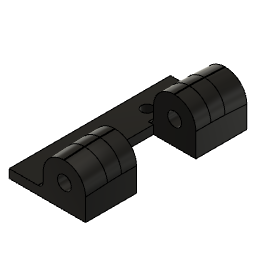
Front mount attachment (Autodesk Fusion 360 design; units mm, degrees)
Autodesk Fusion 360 part; units mm, degrees
box "BoitePrimitive1" add length 25 width 25 height -95 placed x (0, 1, 0) y (-1, 0, 0) z (0, 0, 1) at (25, 0, 0) makes body 1
move_face "DécalerLesFaces3" offset 1.5 1 faces at (16.6667, 25, -63.3333) on bodies 1
sketch "Esquisse8" plane through (0, 0, 0) normal (0, 0, 1) x (1, 0, 0)
  line L0 (0, 0) -> (25, 0)
  line L1 (25, 0) -> (25, 26.5)
  line L2 (25, 26.5) -> (0, 26.5)
  line L3 (0, 26.5) -> (0, 0)
  circle A0 centre (25, 26.5) radius 25 construction
  line L4 (0, 26.5) -> (25, 1.5) construction
  line L5 (25, 26.5) -> (0, 1.5) construction
  point P0 (12.5, 14)
  constraint coincident L1.end L2.start
  constraint coincident L2.end A0
  constraint coincident L2.end L3.start
  constraint coincident A0 L4.end
  constraint coincident L1 L4.end
  constraint coincident L3 L5.end
  constraint perpendicular L4 L5
  constraint midpoint L4 P0
hole "Perçage2" at (12.5, 14, 0) direction (0, 0, -1) diameter 8.2 end through all bodies 1
box "BoitePrimitive2" add length 95 width 20 height 5 placed x (0, 0, -1) y (-1, 0, 0) z (0, 1, 0) at (0, 0, 0) separate body makes body 2
sketch "Esquisse7" plane through (0, 5, 0) normal (0, 1, 0) x (-1, 0, 0)
  line L0 (0, -95) -> (20, -95)
  line L1 (20, -95) -> (20, 0)
  line L2 (20, 0) -> (0, 0)
  line L3 (0, 0) -> (0, -95)
  line L4 (20, -47.5) -> (0, -47.5) construction
  line L5 (20, -95) -> (0, -47.5) construction
  line L6 (0, -47.5) -> (20, 0) construction
  line L7 (0, 0) -> (20, -47.5) construction
  line L8 (20, -47.5) -> (0, -95) construction
  circle A0 centre (10, -71.25) radius 3.3
  circle A1 centre (10, -23.75) radius 3.3
  dimension "d50" = 6.6
  dimension "d51" = 6.6
  constraint midpoint L1 L4.start
  constraint midpoint L3 L4.end
  constraint coincident L0.end L1.start
  constraint coincident L1.end L2.start
  constraint coincident L2.end L3.start
  constraint coincident L0.start L3.end
  constraint midpoint L8 A0.centre
  constraint midpoint L6 A1.centre
  measures "d50" diameter of A0
  measures "d51" diameter of A1
extrude "Extrusion2" cut sketch "Esquisse7" against normal through all contours A0 | A1 bodies 2
combine "Combiner1" operation add target body 1 tool bodies 2
sketch "Esquisse6" plane through (0, 26.5, 0) normal (0, 1, 0) x (-1, 0, 0)
  line L0 (0, -95) -> (0, 0)
  line L1 (0, 0) -> (-25, 0)
  line L2 (-25, 0) -> (-25, -95)
  line L3 (-25, -95) -> (0, -95)
  line L4 (0, -47.5) -> (-25, -47.5) construction
  circle A0 centre (-25, -47.5) radius 17.5 construction
  line L5 (-25, -65) -> (0, -65)
  line L6 (-25, -30) -> (0, -30)
  dimension "d47" = 35
  constraint midpoint L0 L4.start
  constraint midpoint L2 L4.end
  constraint coincident L4.end A0.centre
  constraint coincident A0 L5.start
  constraint coincident L2 L5.start
  constraint coincident L0 L5.end
  constraint tangent A0 L5
  constraint coincident A0 L6.start
  constraint coincident L2 L6.start
  constraint coincident L0 L6.end
  constraint tangent A0 L6
  measures "d47" diameter of A0
extrude "Extrusion1" cut sketch "Esquisse6" against normal through all contours L0 L2 L5 L6 bodies 1
chamfer "Chanfrein1" distance 1 distance2 16.6667 2 edges at (12.5, 26.5, -95) (12.5, 26.5, 0) measured on face at (22.1962, 13.3979, -95) measured on face at (22.1962, 13.3979, 0) on bodies 1
fillet "Congé1" radius 150 2 edges at (12.5, 26.5, -78.3333) (12.5, 26.5, -16.6667) on bodies 1
fillet "Congé2" radius 12.5 6 edges at (25, 26.5, -69.4187) (25, 26.4327, -78.3313) (25, 25.8654, -88.9106) (25, 26.5, -25.5813) (25, 26.4327, -16.6687) (25, 25.8654, -6.0894) on bodies 1
fillet "Congé3" radius 12 6 edges at (0, 25.8654, -88.9106) (0, 26.4327, -78.3313) (0, 26.5, -69.4187) (0, 26.5, -25.5813) (0, 26.4327, -16.6687) (0, 25.8654, -6.0894) on bodies 1
fillet "Congé7" radius 3 2 edges at (0, 5, -15) (0, 5, -80) on bodies 1
equation "planche_larg = 95 mm"
equation "tige_dec = 20 mm"
equation "d3 = base_l"
equation "d4 = base_l"
equation "d5 = -planche_larg"
equation "base_l = 25 mm"
equation "fixation_ep = 5 mm"
equation "fixation_prof = 20 mm"
equation "d11 = planche_larg"
equation "d13 = fixation_ep"
equation "tige_diam = 8 mm"
equation "tige_jeu = 0.2 mm"
equation "vis_diam = 6 mm"
equation "vis_jeu = 0.6 mm"
equation "d26 = base_l / 1.5"
equation "d30 = base_l / 2"
equation "potence_larg = 35 mm"
equation "d47 = potence_larg"
equation "d50 = vis_diam + vis_jeu"
equation "d51 = vis_diam + vis_jeu"
equation "potence_espace = 1.5 mm"
equation "d54 = potence_espace"
equation "d56 = tige_diam + tige_jeu"
named bodies: "Front mount attachment"
